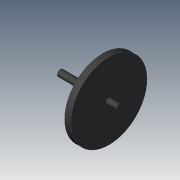
# Autodesk Inventor part: Seal3Dprint
Saved by Autodesk Inventor 2020 (Build 240168000, 168)
## iProperties
Created: 2020-04-10
Part Number: Seal3Dprint
Material: Generic
Document SubType Name: Modeling
Designer: Theo Cominotto
Density: 1 g/cm^3
Appearance: Default
Author: Theo Cominotto
Autodesk Inventor part; units mm, degrees
ref_plane "YZ Plane" through (0, 0, 0) normal (1, 0, 0) x (0, 1, 0)
ref_plane "XZ Plane" through (0, 0, 0) normal (0, 1, 0) x (-1, 0, 0)
ref_plane "XY Plane" through (0, 0, 0) normal (0, 0, 1) x (1, 0, 0)
sketch "Sketch2" plane through (0, 0, 0) normal (0, 0, 1) x (1, 0, 0)
  line L0 (0, 0) -> (0, 1.55)
  line L1 (0, 1.55) -> (20, 1.55)
  line L2 (20, 1.55) -> (20, 18)
  line L3 (20, 18) -> (23, 18)
  line L4 (23, 18) -> (23, 1.35)
  line L5 (23, 1.35) -> (28, 1.35)
  line L6 (28, 1.35) -> (28, 0)
  line L7 (28, 0) -> (0, 0)
  dimension "d3" = 1.55
  dimension "d4" = 20
  dimension "d5" = 3
  dimension "d6" = 5
  dimension "d7" = 1.35
  dimension "d8" = 18
  constraints: 16 end point, 6 perpendicular, 1 horizontal, 1 vertical
  measures "d3" distance of L0.start L0.end
  measures "d4" distance of L0.end L1.end
  measures "d5" distance of L2.end L3.end
  measures "d6" distance of L4.end L5.end
  measures "d7" distance between parallel lines of L7 L5
  measures "d8" distance between parallel lines of L7 L3
revolve "Revolution1" add sketch "Sketch2" angle 360 about axis through (28, 0, 0) along (-1, 0, 0)
body "Solid2"
